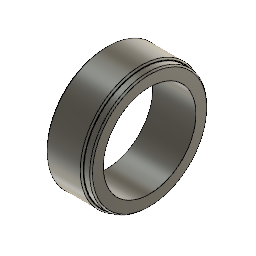
bearing_one_eng_model (Autodesk Fusion 360 design; units mm, degrees)
Autodesk Fusion 360 part; units mm, degrees
sketch "Sketch1" plane through (0, 0, 0) normal (1, 0, 0) x (0, 1, 0)
  circle A0 centre (0, 0) radius 42
  circle A1 centre (0, 0) radius 32
  dimension "d1" = 84
  dimension "d2" = 64
  constraint coincident A0.centre A1.centre
  constraint concentric A0 A1
  measures "d1" diameter of A0
  measures "d2" diameter of A1
extrude "Extrude1" add sketch "Sketch1" along normal blind 25
sketch "Sketch2" plane through (25, 0, 0) normal (1, 0, 0) x (0, 1, 0)
  circle A0 centre (0, 0) radius 32
  circle A1 centre (0, 0) radius 42
  circle A2 centre (0, 0) radius 32
  circle A3 centre (0, 0) radius 40.5
  dimension "d5" = 8.5
  constraint coincident A0.centre A1.centre
  measures "d5" distance of A2 A3
extrude "Extrude2" add sketch "Sketch2" along normal blind 5 contours A3
chamfer "Chamfer1" distance 1 angle 45 3 edges at (0, -39.1577, -15.1878) (25, -39.1577, -15.1878) (30, -37.7593, -14.6454) measured on face at (8.3333, 41.7913, -4.1818) measured on face at (25, 11.2341, 39.8428) measured on face at (30, 37.3967, -3.6019)
